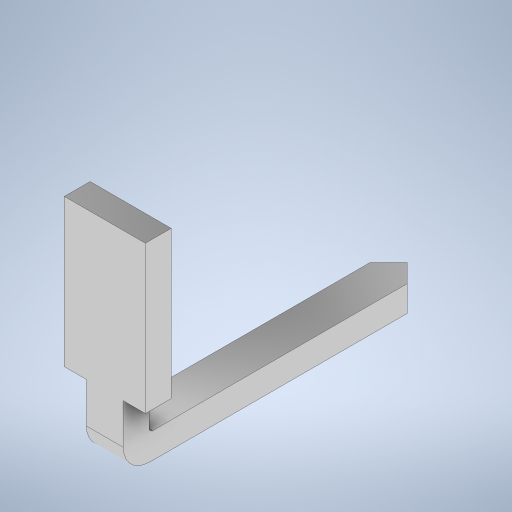
# Autodesk Inventor part: BrueckenGR_LVE2560E_Feet
Saved by Autodesk Inventor 2023.1 (Build 271208000, 208)
## iProperties
Created: 2023-11-19
Part Number: BrueckenGR_LVE2560E_Feet
Material: Nickel-Copper Alloy 400
Document SubType Name: Modeling
Designer: JansenL
Density: 8.83 g/cm^3
Appearance: Chrome - Polished
Author: JansenL
Autodesk Inventor part; units mm, degrees
ref_plane "YZ Plane" through (0, 0, 0) normal (1, 0, 0) x (0, 1, 0)
ref_plane "XZ Plane" through (0, 0, 0) normal (0, 1, 0) x (-1, 0, 0)
ref_plane "XY Plane" through (0, 0, 0) normal (0, 0, 1) x (1, 0, 0)
sketch "Sketch1" plane through (0, 0, 0) normal (0, 0, 1) x (1, 0, 0)
  line L0 (1.1, 0) -> (-1.1, 0)
  line L1 (-1.1, 0) -> (-1.1, -4)
  line L2 (-1.1, -4) -> (-0.5, -4)
  line L3 (-0.5, -4) -> (-0.5, -17)
  line L4 (-0.5, -17) -> (0, -17.5)
  line L5 (0, -17.5) -> (0.5, -17)
  line L6 (0.5, -17) -> (0.5, -4)
  line L7 (0.5, -4) -> (1.1, -4)
  line L8 (1.1, -4) -> (1.1, 0)
  line L9 (0, 0) -> (0, -17.5) construction
  dimension "d0" = 2.2
  dimension "d1" = 17.5
  dimension "d3" = 1
  dimension "d4" = 4
  dimension "d5" = -45
  constraints: 20 end point, 4 perpendicular, 2 equal length, 1 horizontal, 1 midpoint, 1 parallel, 1 vertical, 2 other
  measures "d0" distance between parallel lines of L8 L1
  measures "d1" distance from line of L4.end L0
  measures "d3" distance between parallel lines of L6 L3
  measures "d4" distance between parallel lines of L0 L2
  measures "d5" angle of L4 L3
extrude "Extrusion1" add sketch "Sketch1" along normal blind 0.7
sketch "Sketch2" plane through (0, 0, 0.7) normal (0, 0, 1) x (1, 0, 0)
  line L0 (1.1, 0) -> (-1.1, 0) projected
  line L1 (-0.5, -4) -> (-0.5, -17) projected
  line L2 (0.5, -17) -> (0.5, -4) projected
  point P0 (0, 0)
  point P1 (-0.5, -5)
  point P2 (0.5, -5)
  constraints: 2 point on line
extrude "Extrusion2" [suppressed]
sketch "Sketch3" plane through (0.5, -4, 0.7) normal (1, 0, 0) x (0, 0, -1)
  line L0 (0.7, 0) -> (0.7, -13) projected
  line L1 (0.8, -1.1) -> (8.2, -1.1)
  line L2 (8.2, -1.1) -> (8.2, -1.8)
  line L3 (8.2, -1.8) -> (0.8, -1.8)
  arc A0 (0.7, -1) -> (0.8, -1.1) centre (0.8, -1) ccw
  line L4 (0.7, -13) -> (0.7, 0) projected
  arc A1 (0, -1) -> (0.8, -1.8) centre (0.8, -1) ccw
  line L5 (0, -13) -> (0, 0) projected
  line L6 (0, -1) -> (0.7, -1) projected
  line L7 (0, -1) -> (0.7, -1)
  point P0 (0.7, 4)
  dimension "d12" = 0.7
  dimension "d19" = 0.1
  dimension "d20" = 0.7
  dimension "d21" = 7.5
  constraints: 8 end point, 4 point on circle, 4 tangent, 2 centre point, 2 horizontal, 1 parallel, 1 perpendicular
  measures "d12" distance between parallel lines of L3 L1
  measures "d19" radius of A0
  measures "d20" radial gap between concentric circles of A1 A0
  measures "d21" distance between parallel lines of L2 L0
extrude "Extrusion5" add sketch "Sketch3" against normal blind 1
sketch "Sketch5" plane through (0.5, -5.1, -0.1) normal (0, 1, 0) x (1, 0, 0)
  line L0 (-1, 0) -> (-1, 7.4) projected
  line L1 (-1, 6.9) -> (-0.5, 7.4)
  line L2 (-0.5, 7.4) -> (-1, 7.4)
  line L3 (-1, 7.4) -> (-1, 6.9)
  line L4 (-0.5, 7.4) -> (0, 6.9)
  line L5 (0, 7.4) -> (-1, 7.4) projected
  line L6 (0, 6.9) -> (0, 7.4)
  line L7 (0, 7.4) -> (-0.5, 7.4)
  line L8 (0, 0) -> (-1, 0) construction
  line L9 (-0.5, 0) -> (-0.5, 7.4) construction
  point P0 (-0.5, -0.1)
  dimension "d25" = 90
  constraints: 14 end point, 5 perpendicular, 2 midpoint, 2 point on line, 1 collinear
  measures "d25" angle of L4 L1
extrude "Extrusion6" cut sketch "Sketch5" against normal blind 1
sketch "Sketch6" plane through (0.5, -17, 0.7) normal (1, 0, 0) x (0, 0, -1)
  line L0 (0.7, 0) -> (0.7, 11.2063) projected
  line L1 (0, -0.5) -> (0, 0) projected
  line L2 (0.7, 11.2063) -> (0, 11.2063)
  line L3 (0, 11.2063) -> (0, -0.5)
  line L4 (0, -0.5) -> (0.7, -0.5)
  line L5 (0.7, -0.5) -> (0.7, 11.2063)
  point P0 (0.7, 17)
  constraints: 8 end point, 2 parallel, 1 horizontal, 1 perpendicular
extrude "Extrusion7" cut sketch "Sketch6" against normal blind 10
fillet "Fillet2" radius 0.7 1 edges at (0, -5.7937, 0.7)
body "Solid1"
